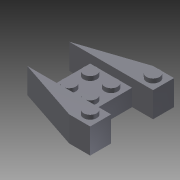
# Autodesk Inventor part: LEGO Brick 2399
Saved by Autodesk Inventor 2011 SP1 (Build 150282100, 282)
## iProperties
Company: Allseas Engineering BV
Created: 2011-09-28
Part Number: LEGO Brick 2399
Cost Center: 0 kg
Material: Steel
Document SubType Name: Modeling
Designer: BvH
Authority: 0 mm^3
Stock Number: =<Filenr>_<Document number>
Density: 7.85 g/cm^3
Act. Code: DW000
SaveDate: 2011-07-28
SaveTime: 18:32
FileName: Standard
TotalMass: 0 kg
TotalVolume: 0 mm^3
Subject: =<Title><TITLE 1_2> <TITLE 2_2>
Author: BvH
Autodesk Inventor part; units mm, degrees
ref_plane "YZ Plane" through (0, 0, 0) normal (1, 0, 0) x (0, 1, 0)
ref_plane "XZ Plane" through (0, 0, 0) normal (0, 1, 0) x (-1, 0, 0)
ref_plane "XY Plane" through (0, 0, 0) normal (0, 0, 1) x (1, 0, 0)
sketch "Sketch1" plane through (0, 0, 0) normal (0, 0, 1) x (1, 0, 0)
  line L0 (0, -22.4) -> (0, 22.4) construction
  line L1 (-22.4, 0) -> (22.4, 0) construction
  line L2 (-16, 16) -> (16, 16)
  line L3 (16, 16) -> (16, -16)
  line L4 (16, -16) -> (-16, -16)
  line L5 (-16, -16) -> (-16, 16)
  line L6 (16, 8) -> (-16, 8)
  line L7 (8, 8) -> (8, -8)
  line L8 (-16, -8) -> (16, -8)
  line L9 (-16, 8) -> (8, 16)
  line L10 (-16, -8) -> (8, -16)
  line L11 (8, -8) -> (16, -16) construction
  line L12 (8, 8) -> (16, 16) construction
  line L13 (-8, 8) -> (-8, -8)
  line L14 (-4, 4) -> (4, 4) construction
  line L15 (4, 4) -> (4, -4) construction
  line L16 (4, -4) -> (-4, -4) construction
  line L17 (-4, -4) -> (-4, 4) construction
  circle A0 centre (-4, 4) radius 2.5
  circle A1 centre (4, 4) radius 2.5
  circle A2 centre (4, -4) radius 2.5
  circle A3 centre (-4, -4) radius 2.5
  circle A4 centre (12, 12) radius 2.5
  circle A5 centre (12, -12) radius 2.5
  line L18 (9.5, -14.5) -> (14.5, -14.5)
  line L19 (14.5, -14.5) -> (14.5, -9.5)
  line L20 (14.5, -9.5) -> (9.5, -9.5)
  line L21 (9.5, -9.5) -> (9.5, -14.5)
  line L22 (9.5, 9.5) -> (14.5, 9.5)
  line L23 (14.5, 9.5) -> (14.5, 14.5)
  line L24 (14.5, 14.5) -> (9.5, 14.5)
  line L25 (9.5, 14.5) -> (9.5, 9.5)
  point P0 (-16, 0)
  point P1 (0, 16)
  point P2 (8, 0)
  point P3 (0, 4)
  point P4 (4, 0)
  dimension "d0" = 32
  dimension "d1" = 32
  dimension "d2" = 8
  dimension "d3" = 16
  dimension "d4" = 16
  dimension "d5" = 8
  dimension "d6" = 5
  constraints: 48 end point, 21 point on line, 8 parallel, 7 midpoint, 6 centre point, 6 horizontal, 5 equal radius, 5 perpendicular, 4 coincident, 4 tangent, 2 vertical
  measures "d0" distance between parallel lines of L4 L2
  measures "d1" distance between parallel lines of L5 L3
  measures "d2" distance between parallel lines of L3 L7
  measures "d3" distance between parallel lines of L8 L6
  measures "d4" distance between parallel lines of L13 L7
  measures "d5" distance of L15.end L16.end
  measures "d6" diameter of A3
extrude "Extrusion1" add sketch "Sketch1" along normal blind 9.6 contours L2 L3 L6 L9 | L8 L3 L4 L10 | A4 | L23 L22 A4 | A4 L24 L23 | A4 L25 L24 | L22 L25 A4 | A5 | L19 L18 A5 | A5 L20 L19 | A5 L21 L20 | L18 L21 A5
extrude "Extrusion5" add sketch "Sketch1" along normal blind 6.4 contours L6 L7 L8 L13 | A0 | A1 | A2 | A3
extrude "Extrusion6" add sketch "Sketch1" along normal blind 8 contours A0 | A1 | A2 | A3
extrude "Extrusion7" add sketch "Sketch1" along normal blind 11.2 contours A4 | A5
extrude "Extrusion8" cut sketch "Sketch1" along normal blind 1.6 contours A4 | L23 L22 A4 | A4 L24 L23 | A4 L25 L24 | L22 L25 A4 | A5 | L19 L18 A5 | A5 L20 L19 | A5 L21 L20 | L18 L21 A5
body "Solid1"
